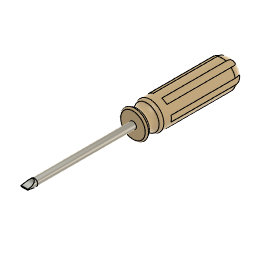
Screw Drive (Autodesk Fusion 360 design; units mm, degrees)
part number: 2025-08-02-17-29-02-179
part number: 2025-08-02-17-49-37-326
part number: 2025-08-02-17-49-51-248
part number: 2025-08-02-18-49-58-994
Autodesk Fusion 360 part; units mm, degrees
sketch "Sketch1" plane through (0, 0, 0) normal (0, 1, 0) x (1, 0, 0) in component " handle"
  circle A0 centre (0, 0) radius 14
  dimension "d1" = 28
  constraint coincident A0.centre origin
  measures "d1" diameter of A0
extrude "Extrude1" add sketch "Sketch1" along normal blind 100 makes body 1 in component " handle"
sketch "Sketch2" plane through (0, 100, 0) normal (0, 1, 0) x (-1, 0, 0) in component " handle"
  circle A0 centre (0, 0) radius 14
  circle A1 centre (-14, 0) radius 3
  dimension "d4" = 6
  constraint coincident A0 A1.centre
  constraint horizontal A0.centre A1.centre
  measures "d4" diameter of A1
extrude "Extrude2" cut sketch "Sketch2" against normal blind 75 contours A0 A1 picked at (-12.9761, 0) bodies 1 in component " handle"
pattern_circular "C-Pattern1" count 6 over 360 about axis through (0, 1.75, 0) along (0, 1, 0) of "Extrude2" in component " handle"
sketch "Sketch3" plane through (0, 0, 0) normal (1, 0, 0) x (0, 1, 0) in component " handle"
  line L0 (0, -14) -> (100, -14)
  line L1 (100, 14) -> (0, 14)
  arc A0 (3, 14) -> (15, 14) centre (9, 17.7466) ccw
  dimension "d9" = 7.0737
  dimension "d10" = 3
  dimension "d11" = 9
  constraint coincident L1 A0.end
  constraint coincident L1 A0.start
  measures "d9" radius of A0
  measures "d10" distance of L1.end A0.start
  measures "d11" horizontal distance of L1.end A0.centre
revolve "Revolve1" cut sketch "Sketch3" angle 360 about axis through (0, 1.75, 0) along (0, 1, 0) bodies 1 in component " handle"
sketch "Sketch4" plane through (0, 0, 0) normal (0, -1, 0) x (1, 0, 0) in component " handle"
  circle A0 centre (0, 0) radius 14
  circle A1 centre (0, 0) radius 3.5
  dimension "d13" = 7
  constraint concentric A0 A1
  measures "d13" diameter of A1
extrude "Extrude3" cut sketch "Sketch4" against normal blind 50 contours A1 bodies 1 in component " handle"
fillet "Fillet1" radius 5 2 edges at (-13.0526, 3, -5.0626) (-13.0526, 15, 5.0626) on bodies 1 in component " handle"
fillet "Fillet1" radius 1.5 1 edges at (-13.0526, 0, 5.0626) on bodies 1 in component " handle"
fillet "Fillet1" radius 10 6 edges at (0, 100, -14) (-12.1244, 100, -7) (-12.1244, 100, 7) (0, 100, 14) (12.1244, 100, 7) (12.1244, 100, -7) on bodies 1 in component " handle"
sketch "Sketch1 (2)" plane through (0, 50, 0) normal (0, -1, 0) x (1, 0, 0) in component "shank"
  circle A0 centre (0, 0) radius 3.5
  circle A1 centre (0, 0) radius 3.5
  circle A2 centre (0, 0) radius 3.5
extrude "Extrude1'" add sketch "Sketch1 (2)" along normal blind 150 separate body makes body 2 in component "shank"
extrude "Extrude1''" add 1 faces at (0.555, -100, -0.9381) along direction (0, -1, 0) blind 10 separate body on bodies 2 makes body 3 in component "tip"
sketch "Sketch1 (3)" plane through (0, 0, 0) normal (1, 0, 0) x (0, 1, 0) in component "tip"
  line L0 (-100, 3.5) -> (-110, 3.5)
  line L1 (-110, -3.5) -> (-100, -3.5)
  arc A0 (-110, 0.5) -> (-101, 3.5) centre (-110.3322, 16.4966) ccw
  line L2 (-110, 0.5) -> (-110, 3.5)
  point P0 (-110, 0)
  dimension "d26" = 0.5
  dimension "d27" = 9
  dimension "d28" = 16
  constraint coincident L0 A0.end
  constraint vertical L0.end A0.start
  constraint coincident L0.end L2.end
  measures "d26" distance of A0.start P0
  measures "d27" distance of L0.end A0.end
  measures "d28" radius of A0
extrude "Extrude2'" cut sketch "Sketch1 (3)" along normal mid plane 20 bodies 3 in component "tip"
mirror "Mirror1" about plane through (0, 0, 0) normal (0, 0, 1) of "Extrude2'" in component "tip"
component " handle" placed x (1, 0, 0) y (0, 1, 0) z (0, 0, 1) at (0, 0, 0)
component "shank" placed x (1, 0, 0) y (0, 1, 0) z (0, 0, 1) at (0, 0, 0)
component "tip" placed x (1, 0, 0) y (0, 1, 0) z (0, 0, 1) at (0, 0, 0)
